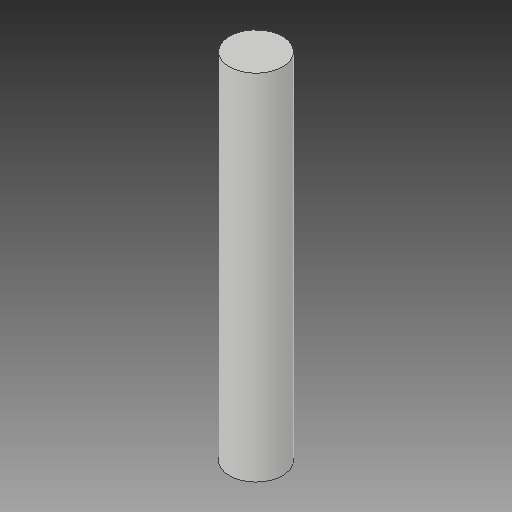
# Autodesk Inventor part: Pin
Saved by Autodesk Inventor 2019 (Build 230136000, 136)
## iProperties
Created: 2018-10-28
Part Number: Pin
Material: Generic
Document SubType Name: Modeling
Designer: Swapnil
Density: 1 g/cm^3
Appearance: Default
Mass: 4.52474 g
Surface Area: 20.4266 cm^2
Volume: 4.52474 cm^3
Author: Swapnil
Autodesk Inventor part; units mm, degrees
ref_plane "YZ Plane" through (0, 0, 0) normal (1, 0, 0) x (0, 1, 0)
ref_plane "XZ Plane" through (0, 0, 0) normal (0, 1, 0) x (-1, 0, 0)
ref_plane "XY Plane" through (0, 0, 0) normal (0, 0, 1) x (1, 0, 0)
sketch "Sketch1" plane through (0, 0, 0) normal (0, 1, 0) x (-1, 0, 0)
  circle A0 centre (0, 0) radius 4.7625
  dimension "d0" = 9.525
  constraints: 1 centre point, 1 coincident
  measures "d0" diameter of A0
extrude "Extrusion1" add sketch "Sketch1" along normal blind 63.5
body "Solid1"
